Autodesk Fusion 360 part; units mm, degrees
(part 11 of 12)
  spline S88 degree 5 poles (70.3993, -3.7669) (70.38, -3.7562) (70.3415, -3.7349) (70.2837, -3.7032) (70.2065, -3.661) (70.1099, -3.6088) (70.0133, -3.5569) (69.9165, -3.5054) (69.8196, -3.4543) (69.7226, -3.4037) (69.6255, -3.3534) (69.5283, -3.3036) (69.431, -3.2541) (69.3336, -3.2051) (69.2361, -3.1565) (69.1385, -3.1083) (69.0408, -3.0606) (68.943, -3.0133) (68.8451, -2.9664) (68.747, -2.9199) (68.6489, -2.8739) (68.5507, -2.8284) (68.4524, -2.7832) (68.3539, -2.7386) (68.2554, -2.6944) (68.1568, -2.6506) (68.0581, -2.6073) (67.9593, -2.5645) (67.8604, -2.5221) (67.7613, -2.4803) (67.6622, -2.4389) (67.563, -2.398) (67.4637, -2.3575) (67.3643, -2.3176) (67.2649, -2.2782) (67.1653, -2.2393) (67.0656, -2.2009) (66.9658, -2.1631) (66.866, -2.1257) (66.766, -2.0889) (66.6659, -2.0527) (66.5658, -2.0169) (66.4656, -1.9818) (66.3652, -1.9472) (66.2648, -1.9132) (66.1643, -1.8797) (66.0637, -1.8469) (65.963, -1.8147) (65.8622, -1.7831) (65.7614, -1.7521) (65.6604, -1.7217) (65.5593, -1.692) (65.4582, -1.663) (65.357, -1.6346) (65.2557, -1.6069) (65.1614, -1.5819) (65.0873, -1.5627) (65.0336, -1.5491) (65.0001, -1.5407) (64.9869, -1.5374) knots -1 -1 -1 -1 -1 -1 -0.985714 -0.971429 -0.957143 -0.942857 -0.928571 -0.914286 -0.9 -0.885714 -0.871429 -0.857143 -0.842857 -0.828571 -0.814286 -0.8 -0.785714 -0.771429 -0.757143 -0.742857 -0.728571 -0.714286 -0.7 -0.685714 -0.671429 -0.657143 -0.642857 -0.628571 -0.614286 -0.6 -0.585714 -0.571429 -0.557143 -0.542857 -0.528571 -0.514286 -0.5 -0.485714 -0.471429 -0.457143 -0.442857 -0.428571 -0.414286 -0.4 -0.385714 -0.371429 -0.357143 -0.342857 -0.328571 -0.314286 -0.3 -0.285714 -0.271429 -0.257143 -0.242857 -0.228571 -0.21931 -0.21931 -0.21931 -0.21931 -0.21931 -0.21931
  spline S89 degree 3 poles (64.9869, -1.5374) (64.7974, -1.4903) (64.6188, -1.4065) (64.304, -1.1753) (64.1706, -1.0301) (63.9972, -0.746) (63.942, -0.6193) (63.8677, -0.3544) (63.849, -0.2175) (63.8491, -0.0799) knots 0 0 0 0 0.058597 0.058597 0.117193 0.117193 0.158456 0.158456 0.199718 0.199718 0.199718 0.199718
  arc A45 (63.8491, -0.0799) -> (63.8491, 0.0799) centre (0, 0) ccw
  spline S90 degree 3 poles (63.8491, 0.0799) (63.8489, 0.2753) (63.8868, 0.4688) (64.0347, 0.8304) (64.1432, 0.995) (64.3767, 1.2322) (64.4862, 1.3165) (64.7252, 1.4528) (64.8534, 1.5042) (64.9869, 1.5374) knots 0 0 0 0 0.058597 0.058597 0.117193 0.117193 0.158456 0.158456 0.199718 0.199718 0.199718 0.199718
  spline S91 degree 5 poles (64.9869, 1.5374) (65.0001, 1.5407) (65.0336, 1.5491) (65.0873, 1.5627) (65.1614, 1.5819) (65.2557, 1.6069) (65.357, 1.6346) (65.4582, 1.663) (65.5593, 1.692) (65.6604, 1.7217) (65.7614, 1.7521) (65.8622, 1.7831) (65.963, 1.8147) (66.0637, 1.8469) (66.1643, 1.8797) (66.2648, 1.9132) (66.3652, 1.9472) (66.4656, 1.9818) (66.5658, 2.0169) (66.6659, 2.0527) (66.766, 2.0889) (66.866, 2.1257) (66.9658, 2.1631) (67.0656, 2.2009) (67.1653, 2.2393) (67.2649, 2.2782) (67.3643, 2.3176) (67.4637, 2.3575) (67.563, 2.398) (67.6622, 2.4389) (67.7613, 2.4803) (67.8604, 2.5221) (67.9593, 2.5645) (68.0581, 2.6073) (68.1568, 2.6506) (68.2554, 2.6944) (68.3539, 2.7386) (68.4524, 2.7832) (68.5507, 2.8284) (68.6489, 2.8739) (68.747, 2.9199) (68.8451, 2.9664) (68.943, 3.0133) (69.0408, 3.0606) (69.1385, 3.1083) (69.2361, 3.1565) (69.3336, 3.2051) (69.431, 3.2541) (69.5283, 3.3036) (69.6255, 3.3534) (69.7226, 3.4037) (69.8196, 3.4543) (69.9165, 3.5054) (70.0133, 3.5569) (70.1099, 3.6088) (70.2065, 3.661) (70.2837, 3.7032) (70.3415, 3.7349) (70.38, 3.7562) (70.3993, 3.7669) knots 0.21931 0.21931 0.21931 0.21931 0.21931 0.21931 0.228571 0.242857 0.257143 0.271429 0.285714 0.3 0.314286 0.328571 0.342857 0.357143 0.371429 0.385714 0.4 0.414286 0.428571 0.442857 0.457143 0.471429 0.485714 0.5 0.514286 0.528571 0.542857 0.557143 0.571429 0.585714 0.6 0.614286 0.628571 0.642857 0.657143 0.671429 0.685714 0.7 0.714286 0.728571 0.742857 0.757143 0.771429 0.785714 0.8 0.814286 0.828571 0.842857 0.857143 0.871429 0.885714 0.9 0.914286 0.928571 0.942857 0.957143 0.971429 0.985714 1 1 1 1 1 1
  arc A46 (70.3993, 3.7669) -> (70.2384, 6.0675) centre (0, 0) ccw
  spline S92 degree 5 poles (70.2384, 6.0675) (70.2179, 6.0754) (70.1768, 6.0911) (70.1151, 6.1145) (70.0328, 6.1455) (69.9299, 6.1838) (69.8269, 6.2217) (69.7239, 6.2592) (69.6209, 6.2963) (69.5178, 6.333) (69.4147, 6.3692) (69.3115, 6.4051) (69.2082, 6.4405) (69.1049, 6.4755) (69.0016, 6.51) (68.8983, 6.5441) (68.7948, 6.5778) (68.6914, 6.6111) (68.5879, 6.6439) (68.4844, 6.6762) (68.3808, 6.7081) (68.2772, 6.7396) (68.1735, 6.7706) (68.0699, 6.8011) (67.9662, 6.8312) (67.8624, 6.8608) (67.7586, 6.8899) (67.6548, 6.9186) (67.551, 6.9467) (67.4471, 6.9744) (67.3432, 7.0016) (67.2393, 7.0283) (67.1353, 7.0545) (67.0313, 7.0802) (66.9273, 7.1054) (66.8233, 7.1301) (66.7192, 7.1542) (66.6152, 7.1778) (66.5111, 7.2009) (66.407, 7.2234) (66.3028, 7.2454) (66.1987, 7.2669) (66.0945, 7.2877) (65.9904, 7.308) (65.8862, 7.3277) (65.782, 7.3469) (65.6778, 7.3654) (65.5736, 7.3833) (65.4694, 7.4005) (65.3652, 7.4172) (65.261, 7.4332) (65.1568, 7.4485) (65.0526, 7.4632) (64.9484, 7.4772) (64.8442, 7.4905) (64.7474, 7.5022) (64.6714, 7.5109) (64.6163, 7.5169) (64.5819, 7.5205) (64.5684, 7.522) knots -1 -1 -1 -1 -1 -1 -0.985714 -0.971429 -0.957143 -0.942857 -0.928571 -0.914286 -0.9 -0.885714 -0.871429 -0.857143 -0.842857 -0.828571 -0.814286 -0.8 -0.785714 -0.771429 -0.757143 -0.742857 -0.728571 -0.714286 -0.7 -0.685714 -0.671429 -0.657143 -0.642857 -0.628571 -0.614286 -0.6 -0.585714 -0.571429 -0.557143 -0.542857 -0.528571 -0.514286 -0.5 -0.485714 -0.471429 -0.457143 -0.442857 -0.428571 -0.414286 -0.4 -0.385714 -0.371429 -0.357143 -0.342857 -0.328571 -0.314286 -0.3 -0.285714 -0.271429 -0.257143 -0.242857 -0.228571 -0.21931 -0.21931 -0.21931 -0.21931 -0.21931 -0.21931
  spline S93 degree 3 poles (64.5684, 7.522) (64.3742, 7.5423) (64.1857, 7.6004) (63.8417, 7.7855) (63.6895, 7.9108) (63.4782, 8.168) (63.4059, 8.2858) (63.2955, 8.5377) (63.2579, 8.6707) (63.2389, 8.8069) knots 0 0 0 0 0.058597 0.058597 0.117193 0.117193 0.158456 0.158456 0.199718 0.199718 0.199718 0.199718
  arc A47 (63.2389, 8.8069) -> (63.2166, 8.9653) centre (0, 0) ccw
  spline S94 degree 3 poles (63.2166, 8.9653) (63.1892, 9.1586) (63.1998, 9.3555) (63.2959, 9.7342) (63.3805, 9.9123) (63.5787, 10.1797) (63.6755, 10.2784) (63.8931, 10.4467) (64.0129, 10.5154) (64.1405, 10.5669) knots 0 0 0 0 0.058597 0.058597 0.117193 0.117193 0.158456 0.158456 0.199718 0.199718 0.199718 0.199718
  spline S95 degree 5 poles (64.1405, 10.5669) (64.1531, 10.572) (64.1851, 10.5849) (64.2364, 10.6059) (64.3071, 10.6352) (64.397, 10.6731) (64.4934, 10.7146) (64.5897, 10.7568) (64.6858, 10.7997) (64.7818, 10.8432) (64.8775, 10.8873) (64.9731, 10.932) (65.0685, 10.9773) (65.1637, 11.0232) (65.2588, 11.0697) (65.3537, 11.1168) (65.4484, 11.1645) (65.5429, 11.2127) (65.6373, 11.2615) (65.7315, 11.3108) (65.8255, 11.3606) (65.9194, 11.411) (66.0131, 11.4618) (66.1066, 11.5132) (66.2, 11.5651) (66.2932, 11.6175) (66.3862, 11.6704) (66.4791, 11.7237) (66.5718, 11.7776) (66.6643, 11.8319) (66.7567, 11.8867) (66.8489, 11.9419) (66.941, 11.9976) (67.0329, 12.0538) (67.1246, 12.1104) (67.2162, 12.1675) (67.3076, 12.225) (67.3988, 12.2829) (67.4899, 12.3412) (67.5809, 12.4) (67.6716, 12.4593) (67.7622, 12.5189) (67.8527, 12.579) (67.9429, 12.6394) (68.0331, 12.7003) (68.123, 12.7616) (68.2128, 12.8233) (68.3024, 12.8854) (68.3919, 12.9479) (68.4812, 13.0108) (68.5704, 13.0741) (68.6594, 13.1377) (68.7482, 13.2018) (68.8369, 13.2662) (68.9254, 13.3311) (69.0138, 13.3963) (69.0843, 13.4487) (69.1371, 13.4882) (69.1723, 13.5147) (69.1899, 13.5279) knots 0.21931 0.21931 0.21931 0.21931 0.21931 0.21931 0.228571 0.242857 0.257143 0.271429 0.285714 0.3 0.314286 0.328571 0.342857 0.357143 0.371429 0.385714 0.4 0.414286 0.428571 0.442857 0.457143 0.471429 0.485714 0.5 0.514286 0.528571 0.542857 0.557143 0.571429 0.585714 0.6 0.614286 0.628571 0.642857 0.657143 0.671429 0.685714 0.7 0.714286 0.728571 0.742857 0.757143 0.771429 0.785714 0.8 0.814286 0.828571 0.842857 0.857143 0.871429 0.885714 0.9 0.914286 0.928571 0.942857 0.957143 0.971429 0.985714 1 1 1 1 1 1
  arc A48 (69.1899, 13.5279) -> (68.7104, 15.7837) centre (0, 0) ccw
  spline S96 degree 5 poles (68.7104, 15.7837) (68.689, 15.7887) (68.6461, 15.7985) (68.5817, 15.8131) (68.4959, 15.8323) (68.3887, 15.856) (68.2815, 15.8792) (68.1743, 15.902) (68.0671, 15.9244) (67.9599, 15.9463) (67.8527, 15.9679) (67.7455, 15.989) (67.6384, 16.0097) (67.5312, 16.03) (67.4241, 16.0498) (67.317, 16.0692) (67.2099, 16.0882) (67.1028, 16.1067) (66.9958, 16.1248) (66.8887, 16.1424) (66.7817, 16.1596) (66.6748, 16.1763) (66.5678, 16.1926) (66.4609, 16.2084) (66.354, 16.2238) (66.2471, 16.2386) (66.1403, 16.253) (66.0335, 16.267) (65.9268, 16.2804) (65.82, 16.2934) (65.7134, 16.3059) (65.6067, 16.3178) (65.5001, 16.3293) (65.3936, 16.3403) (65.2871, 16.3507) (65.1806, 16.3607) (65.0742, 16.3701) (64.9679, 16.379) (64.8616, 16.3874) (64.7554, 16.3952) (64.6492, 16.4025) (64.5431, 16.4092) (64.4371, 16.4154) (64.3311, 16.421) (64.2252, 16.426) (64.1193, 16.4304) (64.0136, 16.4343) (63.9079, 16.4375) (63.8023, 16.4401) (63.6968, 16.4421) (63.5914, 16.4434) (63.4861, 16.4441) (63.3809, 16.4442) (63.2757, 16.4435) (63.1707, 16.4422) (63.0732, 16.4403) (62.9967, 16.4383) (62.9413, 16.4366) (62.9068, 16.4354) (62.8932, 16.4349) knots -1 -1 -1 -1 -1 -1 -0.985714 -0.971429 -0.957143 -0.942857 -0.928571 -0.914286 -0.9 -0.885714 -0.871429 -0.857143 -0.842857 -0.828571 -0.814286 -0.8 -0.785714 -0.771429 -0.757143 -0.742857 -0.728571 -0.714286 -0.7 -0.685714 -0.671429 -0.657143 -0.642857 -0.628571 -0.614286 -0.6 -0.585714 -0.571429 -0.557143 -0.542857 -0.528571 -0.514286 -0.5 -0.485714 -0.471429 -0.457143 -0.442857 -0.428571 -0.414286 -0.4 -0.385714 -0.371429 -0.357143 -0.342857 -0.328571 -0.314286 -0.3 -0.285714 -0.271429 -0.257143 -0.242857 -0.228571 -0.21931 -0.21931 -0.21931 -0.21931 -0.21931 -0.21931
  spline S97 degree 3 poles (62.8932, 16.4349) (62.698, 16.428) (62.5033, 16.4593) (62.1369, 16.5948) (61.9687, 16.6976) (61.7237, 16.9229) (61.6357, 17.0295) (61.4913, 17.2637) (61.4355, 17.3901) (61.3978, 17.5224) knots 0 0 0 0 0.058597 0.058597 0.117193 0.117193 0.158456 0.158456 0.199718 0.199718 0.199718 0.199718
  arc A49 (61.3978, 17.5224) -> (61.3537, 17.6761) centre (0, 0) ccw
  spline S98 degree 3 poles (61.3537, 17.6761) (61.2996, 17.8638) (61.2827, 18.0602) (61.3252, 18.4485) (61.3842, 18.6367) (61.5432, 18.9291) (61.6253, 19.0403) (61.8174, 19.2372) (61.9265, 19.322) (62.0457, 19.3907) knots 0 0 0 0 0.058597 0.058597 0.117193 0.117193 0.158456 0.158456 0.199718 0.199718 0.199718 0.199718
  spline S99 degree 5 poles (62.0457, 19.3907) (62.0574, 19.3975) (62.0873, 19.4148) (62.1352, 19.4427) (62.2011, 19.4815) (62.2848, 19.5316) (62.3746, 19.5861) (62.4641, 19.6413) (62.5533, 19.6971) (62.6422, 19.7535) (62.7309, 19.8105) (62.8194, 19.8681) (62.9075, 19.9262) (62.9954, 19.985) (63.0831, 20.0443) (63.1705, 20.1041) (63.2576, 20.1645) (63.3445, 20.2254) (63.4312, 20.2868) (63.5176, 20.3488) (63.6038, 20.4112) (63.6898, 20.4741) (63.7755, 20.5375) (63.8609, 20.6014) (63.9462, 20.6658) (64.0312, 20.7307) (64.1159, 20.796) (64.2005, 20.8617) (64.2848, 20.928) (64.3689, 20.9946) (64.4527, 21.0617) (64.5364, 21.1293) (64.6198, 21.1973) (64.703, 21.2657) (64.7859, 21.3345) (64.8687, 21.4037) (64.9512, 21.4734) (65.0335, 21.5435) (65.1155, 21.6139) (65.1974, 21.6848) (65.279, 21.7561) (65.3605, 21.8277) (65.4417, 21.8998) (65.5227, 21.9723) (65.6034, 22.0451) (65.684, 22.1183) (65.7643, 22.1919) (65.8444, 22.2659) (65.9243, 22.3402) (66.004, 22.4149) (66.0835, 22.49) (66.1628, 22.5654) (66.2418, 22.6412) (66.3207, 22.7174) (66.3993, 22.7939) (66.4777, 22.8707) (66.5403, 22.9325) (66.5871, 22.979) (66.6183, 23.0101) (66.6339, 23.0256) knots 0.21931 0.21931 0.21931 0.21931 0.21931 0.21931 0.228571 0.242857 0.257143 0.271429 0.285714 0.3 0.314286 0.328571 0.342857 0.357143 0.371429 0.385714 0.4 0.414286 0.428571 0.442857 0.457143 0.471429 0.485714 0.5 0.514286 0.528571 0.542857 0.557143 0.571429 0.585714 0.6 0.614286 0.628571 0.642857 0.657143 0.671429 0.685714 0.7 0.714286 0.728571 0.742857 0.757143 0.771429 0.785714 0.8 0.814286 0.828571 0.842857 0.857143 0.871429 0.885714 0.9 0.914286 0.928571 0.942857 0.957143 0.971429 0.985714 1 1 1 1 1 1
  arc A50 (66.6339, 23.0256) -> (65.8451, 25.1928) centre (0, 0) ccw
  spline S100 degree 5 poles (65.8451, 25.1928) (65.8231, 25.1947) (65.7793, 25.1984) (65.7135, 25.2039) (65.6259, 25.211) (65.5164, 25.2195) (65.407, 25.2276) (65.2977, 25.2352) (65.1884, 25.2425) (65.0792, 25.2493) (64.9701, 25.2558) (64.861, 25.2618) (64.752, 25.2673) (64.6431, 25.2725) (64.5342, 25.2772) (64.4254, 25.2815) (64.3168, 25.2854) (64.2081, 25.2889) (64.0996, 25.2919) (63.9912, 25.2944) (63.8828, 25.2966) (63.7746, 25.2982) (63.6664, 25.2995) (63.5583, 25.3002) (63.4503, 25.3006) (63.3424, 25.3004) (63.2346, 25.2998) (63.127, 25.2988) (63.0194, 25.2972) (62.9119, 25.2952) (62.8045, 25.2927) (62.6972, 25.2897) (62.5901, 25.2862) (62.4831, 25.2823) (62.3761, 25.2778) (62.2693, 25.2729) (62.1627, 25.2674) (62.0561, 25.2614) (61.9497, 25.2549) (61.8434, 25.2479) (61.7373, 25.2403) (61.6312, 25.2322) (61.5254, 25.2235) (61.4197, 25.2143) (61.3141, 25.2046) (61.2087, 25.1942) (61.1034, 25.1833) (60.9983, 25.1718) (60.8934, 25.1597) (60.7886, 25.1469) (60.6841, 25.1336) (60.5797, 25.1196) (60.4755, 25.105) (60.3714, 25.0898) (60.2676, 25.0739) (60.1713, 25.0584) (60.0959, 25.0458) (60.0412, 25.0364) (60.0072, 25.0304) (59.9938, 25.028) knots -1 -1 -1 -1 -1 -1 -0.985714 -0.971429 -0.957143 -0.942857 -0.928571 -0.914286 -0.9 -0.885714 -0.871429 -0.857143 -0.842857 -0.828571 -0.814286 -0.8 -0.785714 -0.771429 -0.757143 -0.742857 -0.728571 -0.714286 -0.7 -0.685714 -0.671429 -0.657143 -0.642857 -0.628571 -0.614286 -0.6 -0.585714 -0.571429 -0.557143 -0.542857 -0.528571 -0.514286 -0.5 -0.485714 -0.471429 -0.457143 -0.442857 -0.428571 -0.414286 -0.4 -0.385714 -0.371429 -0.357143 -0.342857 -0.328571 -0.314286 -0.3 -0.285714 -0.271429 -0.257143 -0.242857 -0.228571 -0.21931 -0.21931 -0.21931 -0.21931 -0.21931 -0.21931
  spline S101 degree 3 poles (59.9938, 25.028) (59.8015, 24.994) (59.6043, 24.9979) (59.2226, 25.0811) (59.0417, 25.1595) (58.7677, 25.3485) (58.6658, 25.4418) (58.4902, 25.6536) (58.4174, 25.771) (58.3616, 25.8968) knots 0 0 0 0 0.058597 0.058597 0.117193 0.117193 0.158456 0.158456 0.199718 0.199718 0.199718 0.199718
  arc A51 (58.3616, 25.8968) -> (58.2966, 26.0428) centre (0, 0) ccw
  spline S102 degree 3 poles (58.2966, 26.0428) (58.2169, 26.2212) (58.1728, 26.4134) (58.1608, 26.8038) (58.193, 26.9983) (58.3099, 27.31) (58.3757, 27.4316) (58.5385, 27.6533) (58.6347, 27.7524) (58.7432, 27.8371) knots 0 0 0 0 0.058597 0.058597 0.117193 0.117193 0.158456 0.158456 0.199718 0.199718 0.199718 0.199718
  spline S103 degree 5 poles (58.7432, 27.8371) (58.7539, 27.8454) (58.781, 27.8667) (58.8246, 27.901) (58.8845, 27.9486) (58.9604, 28.0099) (59.0417, 28.0764) (59.1226, 28.1435) (59.2032, 28.2111) (59.2835, 28.2794) (59.3634, 28.3482) (59.4429, 28.4175) (59.5221, 28.4874) (59.601, 28.5578) (59.6795, 28.6287) (59.7578, 28.7001) (59.8357, 28.772) (59.9133, 28.8444) (59.9905, 28.9173) (60.0675, 28.9907) (60.1441, 29.0645) (60.2205, 29.1388) (60.2965, 29.2135) (60.3723, 29.2887) (60.4477, 29.3643) (60.5229, 29.4403) (60.5977, 29.5168) (60.6723, 29.5937) (60.7466, 29.671) (60.8206, 29.7487) (60.8943, 29.8269) (60.9677, 29.9054) (61.0408, 29.9843) (61.1137, 30.0636) (61.1862, 30.1433) (61.2585, 30.2234) (61.3306, 30.3039) (61.4023, 30.3847) (61.4738, 30.4659) (61.545, 30.5475) (61.6159, 30.6294) (61.6865, 30.7117) (61.7569, 30.7944) (61.827, 30.8774) (61.8969, 30.9608) (61.9665, 31.0445) (62.0358, 31.1285) (62.1048, 31.2129) (62.1736, 31.2977) (62.2421, 31.3828) (62.3104, 31.4682) (62.3784, 31.5539) (62.4461, 31.64) (62.5136, 31.7263) (62.5808, 31.813) (62.6478, 31.9001) (62.7011, 31.97) (62.741, 32.0225) (62.7676, 32.0576) (62.7808, 32.0752) knots 0.21931 0.21931 0.21931 0.21931 0.21931 0.21931 0.228571 0.242857 0.257143 0.271429 0.285714 0.3 0.314286 0.328571 0.342857 0.357143 0.371429 0.385714 0.4 0.414286 0.428571 0.442857 0.457143 0.471429 0.485714 0.5 0.514286 0.528571 0.542857 0.557143 0.571429 0.585714 0.6 0.614286 0.628571 0.642857 0.657143 0.671429 0.685714 0.7 0.714286 0.728571 0.742857 0.757143 0.771429 0.785714 0.8 0.814286 0.828571 0.842857 0.857143 0.871429 0.885714 0.9 0.914286 0.928571 0.942857 0.957143 0.971429 0.985714 1 1 1 1 1 1
  arc A52 (62.7808, 32.0752) -> (61.6981, 34.1115) centre (0, 0) ccw
  spline S104 degree 5 poles (61.6981, 34.1115) (61.6761, 34.1103) (61.6322, 34.1079) (61.5663, 34.1042) (61.4785, 34.0991) (61.369, 34.0922) (61.2595, 34.085) (61.1501, 34.0773) (61.0409, 34.0693) (60.9318, 34.0609) (60.8228, 34.0521) (60.714, 34.0428) (60.6053, 34.0332) (60.4967, 34.0231) (60.3883, 34.0127) (60.2799, 34.0018) (60.1718, 33.9905) (60.0637, 33.9788) (59.9559, 33.9667) (59.8481, 33.9541) (59.7405, 33.9411) (59.6331, 33.9277) (59.5258, 33.9139) (59.4187, 33.8996) (59.3117, 33.8849) (59.2049, 33.8698) (59.0982, 33.8542) (58.9917, 33.8381) (58.8854, 33.8216) (58.7792, 33.8047) (58.6732, 33.7872) (58.5674, 33.7694) (58.4618, 33.751) (58.3564, 33.7322) (58.2511, 33.7129) (58.146, 33.6931) (58.0412, 33.6729) (57.9365, 33.6521) (57.832, 33.6308) (57.7277, 33.6091) (57.6237, 33.5868) (57.5198, 33.564) (57.4162, 33.5407) (57.3128, 33.5169) (57.2096, 33.4925) (57.1066, 33.4676) (57.0039, 33.4422) (56.9014, 33.4161) (56.7992, 33.3895) (56.6973, 33.3624) (56.5956, 33.3346) (56.4941, 33.3062) (56.393, 33.2773) (56.2921, 33.2477) (56.1915, 33.2175) (56.0983, 33.1888) (56.0253, 33.1658) (55.9725, 33.1488) (55.9396, 33.1382) (55.9267, 33.134) knots -1 -1 -1 -1 -1 -1 -0.985714 -0.971429 -0.957143 -0.942857 -0.928571 -0.914286 -0.9 -0.885714 -0.871429 -0.857143 -0.842857 -0.828571 -0.814286 -0.8 -0.785714 -0.771429 -0.757143 -0.742857 -0.728571 -0.714286 -0.7 -0.685714 -0.671429 -0.657143 -0.642857 -0.628571 -0.614286 -0.6 -0.585714 -0.571429 -0.557143 -0.542857 -0.528571 -0.514286 -0.5 -0.485714 -0.471429 -0.457143 -0.442857 -0.428571 -0.414286 -0.4 -0.385714 -0.371429 -0.357143 -0.342857 -0.328571 -0.314286 -0.3 -0.285714 -0.271429 -0.257143 -0.242857 -0.228571 -0.21931 -0.21931 -0.21931 -0.21931 -0.21931 -0.21931
  spline S105 degree 3 poles (55.9267, 33.134) (55.741, 33.0736) (55.5452, 33.05) (55.1557, 33.0792) (54.9656, 33.1317) (54.668, 33.2807) (54.5541, 33.3589) (54.3507, 33.5442) (54.2623, 33.6504) (54.1895, 33.7671) knots 0 0 0 0 0.058597 0.058597 0.117193 0.117193 0.158456 0.158456 0.199718 0.199718 0.199718 0.199718
  arc A53 (54.1895, 33.7671) -> (54.1048, 33.9027) centre (0, 0) ccw
  spline S106 degree 3 poles (54.1048, 33.9027) (54.0011, 34.0682) (53.9307, 34.2524) (53.8645, 34.6374) (53.8693, 34.8345) (53.9416, 35.1594) (53.9898, 35.2889) (54.1202, 35.5312) (54.2017, 35.6427) (54.2973, 35.7416) knots 0 0 0 0 0.058597 0.058597 0.117193 0.117193 0.158456 0.158456 0.199718 0.199718 0.199718 0.199718
  spline S107 degree 5 poles (54.2973, 35.7416) (54.3067, 35.7514) (54.3307, 35.7762) (54.3691, 35.8163) (54.4217, 35.8718) (54.4884, 35.943) (54.5597, 36.0202) (54.6305, 36.0979) (54.7008, 36.1761) (54.7708, 36.2548) (54.8403, 36.3341) (54.9095, 36.4138) (54.9782, 36.494) (55.0465, 36.5747) (55.1144, 36.6558) (55.1819, 36.7375) (55.2491, 36.8195) (55.3158, 36.902) (55.3822, 36.985) (55.4482, 37.0683) (55.5138, 37.1521) (55.5791, 37.2363) (55.644, 37.3209) (55.7085, 37.4058) (55.7727, 37.4912) (55.8366, 37.577) (55.9, 37.6631) (55.9632, 37.7496) (56.026, 37.8365) (56.0884, 37.9238) (56.1505, 38.0114) (56.2123, 38.0994) (56.2738, 38.1877) (56.3349, 38.2764) (56.3956, 38.3654) (56.4561, 38.4548) (56.5162, 38.5445) (56.576, 38.6346) (56.6355, 38.7249) (56.6946, 38.8156) (56.7535, 38.9066) (56.812, 38.998) (56.8702, 39.0896) (56.928, 39.1816) (56.9856, 39.2739) (57.0429, 39.3664) (57.0998, 39.4593) (57.1564, 39.5525) (57.2127, 39.646) (57.2688, 39.7398) (57.3245, 39.8338) (57.3799, 39.9282) (57.435, 40.0229) (57.4898, 40.1178) (57.5443, 40.213) (57.5985, 40.3085) (57.6416, 40.3851) (57.6738, 40.4427) (57.6952, 40.4812) (57.7059, 40.5004) knots 0.21931 0.21931 0.21931 0.21931 0.21931 0.21931 0.228571 0.242857 0.257143 0.271429 0.285714 0.3 0.314286 0.328571 0.342857 0.357143 0.371429 0.385714 0.4 0.414286 0.428571 0.442857 0.457143 0.471429 0.485714 0.5 0.514286 0.528571 0.542857 0.557143 0.571429 0.585714 0.6 0.614286 0.628571 0.642857 0.657143 0.671429 0.685714 0.7 0.714286 0.728571 0.742857 0.757143 0.771429 0.785714 0.8 0.814286 0.828571 0.842857 0.857143 0.871429 0.885714 0.9 0.914286 0.928571 0.942857 0.957143 0.971429 0.985714 1 1 1 1 1 1
  arc A54 (57.7059, 40.5004) -> (56.3503, 42.3662) centre (0, 0) ccw
  spline S108 degree 5 poles (56.3503, 42.3662) (56.3287, 42.362) (56.2855, 42.3535) (56.2208, 42.3407) (56.1346, 42.3234) (56.027, 42.3013) (55.9196, 42.2789) (55.8124, 42.2562) (55.7053, 42.233) (55.5985, 42.2095) (55.4918, 42.1856) (55.3853, 42.1613) (55.279, 42.1366) (55.1729, 42.1115) (55.0669, 42.0861) (54.9612, 42.0602) (54.8556, 42.034) (54.7503, 42.0074) (54.6451, 41.9804) (54.5402, 41.9529) (54.4354, 41.9251) (54.3309, 41.8969) (54.2266, 41.8682) (54.1225, 41.8392) (54.0186, 41.8097) (53.9149, 41.7799) (53.8115, 41.7496) (53.7082, 41.7189) (53.6052, 41.6877) (53.5025, 41.6562) (53.4, 41.6242) (53.2977, 41.5917) (53.1956, 41.5589) (53.0938, 41.5256) (52.9923, 41.4918) (52.891, 41.4576) (52.79, 41.4229) (52.6892, 41.3878) (52.5887, 41.3522) (52.4884, 41.3162) (52.3885, 41.2796) (52.2888, 41.2426) (52.1894, 41.2051) (52.0903, 41.1671) (51.9916, 41.1286) (51.8931, 41.0896) (51.7949, 41.0501) (51.697, 41.0101) (51.5995, 40.9695) (51.5023, 40.9284) (51.4055, 40.8868) (51.309, 40.8446) (51.2129, 40.8018) (51.1171, 40.7585) (51.0217, 40.7146) (50.9333, 40.6731) (50.8643, 40.6402) (50.8143, 40.6161) (50.7833, 40.601) (50.7711, 40.595) knots -1 -1 -1 -1 -1 -1 -0.985714 -0.971429 -0.957143 -0.942857 -0.928571 -0.914286 -0.9 -0.885714 -0.871429 -0.857143 -0.842857 -0.828571 -0.814286 -0.8 -0.785714 -0.771429 -0.757143 -0.742857 -0.728571 -0.714286 -0.7 -0.685714 -0.671429 -0.657143 -0.642857 -0.628571 -0.614286 -0.6 -0.585714 -0.571429 -0.557143 -0.542857 -0.528571 -0.514286 -0.5 -0.485714 -0.471429 -0.457143 -0.442857 -0.428571 -0.414286 -0.4 -0.385714 -0.371429 -0.357143 -0.342857 -0.328571 -0.314286 -0.3 -0.285714 -0.271429 -0.257143 -0.242857 -0.228571 -0.21931 -0.21931 -0.21931 -0.21931 -0.21931 -0.21931
  spline S109 degree 3 poles (50.7711, 40.595) (50.5956, 40.5093) (50.405, 40.4587) (50.0152, 40.4334) (49.8197, 40.459) (49.5042, 40.5651) (49.3805, 40.6267) (49.1533, 40.7819) (49.051, 40.8747) (48.9627, 40.9802) knots 0 0 0 0 0.058597 0.058597 0.117193 0.117193 0.158456 0.158456 0.199718 0.199718 0.199718 0.199718
  arc A55 (48.9627, 40.9802) -> (48.8599, 41.1027) centre (0, 0) ccw
  spline S110 degree 3 poles (48.8599, 41.1027) (48.7342, 41.2522) (48.6388, 41.4248) (48.5197, 41.7968) (48.497, 41.9927) (48.5234, 42.3245) (48.5531, 42.4594) (48.6485, 42.7174) (48.7137, 42.8393) (48.7946, 42.9505) knots 0 0 0 0 0.058597 0.058597 0.117193 0.117193 0.158456 0.158456 0.199718 0.199718 0.199718 0.199718
  spline S111 degree 5 poles (48.7946, 42.9505) (48.8026, 42.9615) (48.8229, 42.9894) (48.8553, 43.0345) (48.8997, 43.0967) (48.9558, 43.1765) (49.0156, 43.2629) (49.0749, 43.3497) (49.1338, 43.4369) (49.1921, 43.5246) (49.2499, 43.6128) (49.3073, 43.7013) (49.3642, 43.7903) (49.4206, 43.8797) (49.4765, 43.9696) (49.532, 44.0598) (49.5871, 44.1504) (49.6417, 44.2414) (49.6959, 44.3327) (49.7497, 44.4245) (49.803, 44.5166) (49.8559, 44.609) (49.9084, 44.7018) (49.9605, 44.7949) (50.0122, 44.8884) (50.0635, 44.9822) (50.1143, 45.0764) (50.1648, 45.1708) (50.2149, 45.2656) (50.2646, 45.3607) (50.3139, 45.4561) (50.3629, 45.5519) (50.4114, 45.6479) (50.4596, 45.7442) (50.5074, 45.8408) (50.5548, 45.9377) (50.6018, 46.0349) (50.6485, 46.1324) (50.6948, 46.2302) (50.7408, 46.3282) (50.7864, 46.4265) (50.8316, 46.5251) (50.8765, 46.624) (50.921, 46.7231) (50.9652, 46.8225) (51.009, 46.9222) (51.0524, 47.0221) (51.0955, 47.1222) (51.1383, 47.2226) (51.1807, 47.3233) (51.2228, 47.4242) (51.2645, 47.5254) (51.3059, 47.6268) (51.347, 47.7284) (51.3877, 47.8303) (51.428, 47.9324) (51.4601, 48.0143) (51.4839, 48.0758) (51.4998, 48.1168) (51.5077, 48.1374) knots 0.21931 0.21931 0.21931 0.21931 0.21931 0.21931 0.228571 0.242857 0.257143 0.271429 0.285714 0.3 0.314286 0.328571 0.342857 0.357143 0.371429 0.385714 0.4 0.414286 0.428571 0.442857 0.457143 0.471429 0.485714 0.5 0.514286 0.528571 0.542857 0.557143 0.571429 0.585714 0.6 0.614286 0.628571 0.642857 0.657143 0.671429 0.685714 0.7 0.714286 0.728571 0.742857 0.757143 0.771429 0.785714 0.8 0.814286 0.828571 0.842857 0.857143 0.871429 0.885714 0.9 0.914286 0.928571 0.942857 0.957143 0.971429 0.985714 1 1 1 1 1 1
  arc A56 (51.5077, 48.1374) -> (49.9056, 49.7964) centre (0, 0) ccw
  spline S112 degree 5 poles (49.9056, 49.7964) (49.8848, 49.7892) (49.8433, 49.7748) (49.7809, 49.7531) (49.698, 49.7239) (49.5945, 49.6871) (49.4913, 49.65) (49.3883, 49.6125) (49.2855, 49.5747) (49.183, 49.5365) (49.0807, 49.498) (48.9786, 49.4591) (48.8767, 49.4199) (48.7751, 49.3803) (48.6738, 49.3403) (48.5726, 49.3) (48.4718, 49.2594) (48.3712, 49.2183) (48.2708, 49.1769) (48.1707, 49.1352) (48.0708, 49.093) (47.9712, 49.0505) (47.8719, 49.0077) (47.7729, 48.9644) (47.6741, 48.9208) (47.5756, 48.8768) (47.4774, 48.8324) (47.3794, 48.7876) (47.2818, 48.7424) (47.1844, 48.6969) (47.0873, 48.6509) (46.9905, 48.6046) (46.8941, 48.5578) (46.7979, 48.5107) (46.702, 48.4631) (46.6065, 48.4151) (46.5112, 48.3667) (46.4163, 48.3179) (46.3218, 48.2687) (46.2275, 48.219) (46.1336, 48.169) (46.0401, 48.1184) (45.9469, 48.0675) (45.8541, 48.0161) (45.7616, 47.9642) (45.6695, 47.9119) (45.5778, 47.8591) (45.4864, 47.8058) (45.3955, 47.7521) (45.305, 47.6978) (45.2149, 47.6431) (45.1252, 47.5879) (45.0359, 47.5322) (44.9471, 47.4759) (44.8588, 47.4192) (44.7771, 47.3659) (44.7133, 47.3237) (44.6671, 47.2928) (44.6385, 47.2735) (44.6273, 47.2659) knots -1 -1 -1 -1 -1 -1 -0.985714 -0.971429 -0.957143 -0.942857 -0.928571 -0.914286 -0.9 -0.885714 -0.871429 -0.857143 -0.842857 -0.828571 -0.814286 -0.8 -0.785714 -0.771429 -0.757143 -0.742857 -0.728571 -0.714286 -0.7 -0.685714 -0.671429 -0.657143 -0.642857 -0.628571 -0.614286 -0.6 -0.585714 -0.571429 -0.557143 -0.542857 -0.528571 -0.514286 -0.5 -0.485714 -0.471429 -0.457143 -0.442857 -0.428571 -0.414286 -0.4 -0.385714 -0.371429 -0.357143 -0.342857 -0.328571 -0.314286 -0.3 -0.285714 -0.271429 -0.257143 -0.242857 -0.228571 -0.21931 -0.21931 -0.21931 -0.21931 -0.21931 -0.21931
  spline S113 degree 3 poles (44.6273, 47.2659) (44.4654, 47.1566) (44.2837, 47.08) (43.9012, 47.0007) (43.704, 46.9988) (43.3768, 47.06) (43.2458, 47.1038) (42.9992, 47.2258) (42.8849, 47.3035) (42.7828, 47.3957) knots 0 0 0 0 0.058597 0.058597 0.117193 0.117193 0.158456 0.158456 0.199718 0.199718 0.199718 0.199718
  arc A57 (42.7828, 47.3957) -> (42.664, 47.5027) centre (0, 0) ccw
  spline S114 degree 3 poles (42.664, 47.5027) (42.5187, 47.6332) (42.4003, 47.7908) (42.2305, 48.1426) (42.1808, 48.3335) (42.1607, 48.6657) (42.1714, 48.8035) (42.2299, 49.0723) (42.2776, 49.202) (42.3422, 49.3234) knots 0 0 0 0 0.058597 0.058597 0.117193 0.117193 0.158456 0.158456 0.199718 0.199718 0.199718 0.199718
  spline S115 degree 5 poles (42.3422, 49.3234) (42.3486, 49.3354) (42.3648, 49.3659) (42.3906, 49.415) (42.4259, 49.4828) (42.4704, 49.5697) (42.5176, 49.6635) (42.5642, 49.7577) (42.6103, 49.8523) (42.6559, 49.9473) (42.7009, 50.0426) (42.7454, 50.1383) (42.7893, 50.2343) (42.8327, 50.3307) (42.8756, 50.4274) (42.9181, 50.5245) (42.96, 50.6219) (43.0014, 50.7196) (43.0423, 50.8176) (43.0828, 50.9159) (43.1228, 51.0146) (43.1623, 51.1135) (43.2014, 51.2127) (43.24, 51.3122) (43.2782, 51.4119) (43.3159, 51.512) (43.3532, 51.6123) (43.3901, 51.7128) (43.4265, 51.8137) (43.4624, 51.9148) (43.498, 52.0161) (43.5331, 52.1177) (43.5678, 52.2196) (43.6021, 52.3216) (43.636, 52.424) (43.6695, 52.5265) (43.7026, 52.6293) (43.7352, 52.7324) (43.7675, 52.8356) (43.7993, 52.9391) (43.8308, 53.0428) (43.8619, 53.1467) (43.8926, 53.2509) (43.9228, 53.3552) (43.9527, 53.4598) (43.9823, 53.5646) (44.0114, 53.6696) (44.0401, 53.7748) (44.0685, 53.8801) (44.0965, 53.9857) (44.1241, 54.0915) (44.1514, 54.1975) (44.1782, 54.3037) (44.2047, 54.41) (44.2309, 54.5166) (44.2567, 54.6233) (44.277, 54.7089) (44.2921, 54.7731) (44.302, 54.8159) (44.307, 54.8374) knots 0.21931 0.21931 0.21931 0.21931 0.21931 0.21931 0.228571 0.242857 0.257143 0.271429 0.285714 0.3 0.314286 0.328571 0.342857 0.357143 0.371429 0.385714 0.4 0.414286 0.428571 0.442857 0.457143 0.471429 0.485714 0.5 0.514286 0.528571 0.542857 0.557143 0.571429 0.585714 0.6 0.614286 0.628571 0.642857 0.657143 0.671429 0.685714 0.7 0.714286 0.728571 0.742857 0.757143 0.771429 0.785714 0.8 0.814286 0.828571 0.842857 0.857143 0.871429 0.885714 0.9 0.914286 0.928571 0.942857 0.957143 0.971429 0.985714 1 1 1 1 1 1
  arc A58 (44.307, 54.8374) -> (42.4897, 56.2573) centre (0, 0) ccw
  spline S116 degree 5 poles (42.4897, 56.2573) (42.4701, 56.2473) (42.4309, 56.2272) (42.3722, 56.197) (42.2941, 56.1566) (42.1968, 56.1058) (42.0997, 56.0547) (42.0029, 56.0032) (41.9064, 55.9514) (41.8102, 55.8994) (41.7142, 55.847) (41.6185, 55.7943) (41.5231, 55.7412) (41.428, 55.6879) (41.3332, 55.6342) (41.2387, 55.5803) (41.1445, 55.5259) (41.0505, 55.4713) (40.9569, 55.4164) (40.8636, 55.3611) (40.7706, 55.3054) (40.6779, 55.2495) (40.5855, 55.1932) (40.4934, 55.1366) (40.4017, 55.0796) (40.3103, 55.0224) (40.2192, 54.9647) (40.1284, 54.9067) (40.038, 54.8484) (39.9479, 54.7898) (39.8582, 54.7307) (39.7688, 54.6714) (39.6797, 54.6117) (39.5911, 54.5516) (39.5028, 54.4911) (39.4148, 54.4303) (39.3273, 54.3692) (39.2401, 54.3076) (39.1533, 54.2457) (39.0669, 54.1834) (38.9808, 54.1207) (38.8952, 54.0577) (38.81, 53.9943) (38.7253, 53.9304) (38.6409, 53.8662) (38.557, 53.8016) (38.4735, 53.7365) (38.3905, 53.6711) (38.3079, 53.6052) (38.2258, 53.5389) (38.1442, 53.4721) (38.0631, 53.405) (37.9825, 53.3374) (37.9023, 53.2693) (37.8227, 53.2008) (37.7492, 53.1367) (37.6919, 53.086) (37.6506, 53.049) (37.6249, 53.026) (37.6148, 53.0169) knots -1 -1 -1 -1 -1 -1 -0.985714 -0.971429 -0.957143 -0.942857 -0.928571 -0.914286 -0.9 -0.885714 -0.871429 -0.857143 -0.842857 -0.828571 -0.814286 -0.8 -0.785714 -0.771429 -0.757143 -0.742857 -0.728571 -0.714286 -0.7 -0.685714 -0.671429 -0.657143 -0.642857 -0.628571 -0.614286 -0.6 -0.585714 -0.571429 -0.557143 -0.542857 -0.528571 -0.514286 -0.5 -0.485714 -0.471429 -0.457143 -0.442857 -0.428571 -0.414286 -0.4 -0.385714 -0.371429 -0.357143 -0.342857 -0.328571 -0.314286 -0.3 -0.285714 -0.271429 -0.257143 -0.242857 -0.228571 -0.21931 -0.21931 -0.21931 -0.21931 -0.21931 -0.21931
  spline S117 degree 3 poles (37.6148, 53.0169) (37.4697, 52.8861) (37.3005, 52.7849) (36.9327, 52.6532) (36.7377, 52.6238) (36.4052, 52.6389) (36.2693, 52.664) (36.0082, 52.7506) (35.8842, 52.8116) (35.7703, 52.8886) knots 0 0 0 0 0.058597 0.058597 0.117193 0.117193 0.158456 0.158456 0.199718 0.199718 0.199718 0.199718
  arc A59 (35.7703, 52.8886) -> (35.6377, 52.9781) centre (0, 0) ccw
  spline S118 degree 3 poles (35.6377, 52.9781) (35.4756, 53.0871) (35.3364, 53.2267) (35.1193, 53.5515) (35.0435, 53.7335) (34.9775, 54.0598) (34.9689, 54.1977) (34.9894, 54.472) (35.0185, 54.6071) (35.0656, 54.7363) knots 0 0 0 0 0.058597 0.058597 0.117193 0.117193 0.158456 0.158456 0.199718 0.199718 0.199718 0.199718
  spline S119 degree 5 poles (35.0656, 54.7363) (35.0703, 54.7491) (35.0821, 54.7815) (35.1008, 54.8337) (35.1264, 54.9058) (35.1583, 54.998) (35.192, 55.0975) (35.2251, 55.1973) (35.2576, 55.2973) (35.2894, 55.3977) (35.3207, 55.4984) (35.3515, 55.5993) (35.3816, 55.7006) (35.4112, 55.8021) (35.4402, 55.9038) (35.4687, 56.0059) (35.4967, 56.1081) (35.5241, 56.2106) (35.551, 56.3134) (35.5774, 56.4164) (35.6033, 56.5196) (35.6287, 56.6231) (35.6536, 56.7267) (35.678, 56.8306) (35.7019, 56.9347) (35.7253, 57.0391) (35.7483, 57.1436) (35.7708, 57.2483) (35.7928, 57.3532) (35.8143, 57.4583) (35.8354, 57.5636) (35.8561, 57.6691) (35.8763, 57.7748) (35.896, 57.8807) (35.9154, 57.9868) (35.9342, 58.093) (35.9527, 58.1994) (35.9707, 58.306) (35.9882, 58.4127) (36.0054, 58.5196) (36.0221, 58.6267) (36.0384, 58.7339) (36.0543, 58.8413) (36.0698, 58.9489) (36.0848, 59.0566) (36.0995, 59.1644) (36.1137, 59.2725) (36.1275, 59.3806) (36.141, 59.4889) (36.154, 59.5974) (36.1666, 59.706) (36.1789, 59.8147) (36.1907, 59.9236) (36.2021, 60.0326) (36.2132, 60.1418) (36.2239, 60.2511) (36.2321, 60.3386) (36.2381, 60.4043) (36.242, 60.4481) (36.2439, 60.4701) knots 0.21931 0.21931 0.21931 0.21931 0.21931 0.21931 0.228571 0.242857 0.257143 0.271429 0.285714 0.3 0.314286 0.328571 0.342857 0.357143 0.371429 0.385714 0.4 0.414286 0.428571 0.442857 0.457143 0.471429 0.485714 0.5 0.514286 0.528571 0.542857 0.557143 0.571429 0.585714 0.6 0.614286 0.628571 0.642857 0.657143 0.671429 0.685714 0.7 0.714286 0.728571 0.742857 0.757143 0.771429 0.785714 0.8 0.814286 0.828571 0.842857 0.857143 0.871429 0.885714 0.9 0.914286 0.928571 0.942857 0.957143 0.971429 0.985714 1 1 1 1 1 1
  arc A60 (36.2439, 60.4701) -> (34.2466, 61.6232) centre (0, 0) ccw
  spline S120 degree 5 poles (34.2466, 61.6232) (34.2286, 61.6105) (34.1926, 61.5852) (34.1387, 61.5472) (34.067, 61.4963) (33.9777, 61.4324) (33.8887, 61.3683) (33.8, 61.3039) (33.7117, 61.2392) (33.6236, 61.1742) (33.5359, 61.109) (33.4484, 61.0435) (33.3614, 60.9777) (33.2746, 60.9116) (33.1882, 60.8453) (33.1021, 60.7787) (33.0163, 60.7118) (32.9309, 60.6446) (32.8459, 60.5771) (32.7611, 60.5094) (32.6768, 60.4414) (32.5928, 60.3731) (32.5091, 60.3045) (32.4258, 60.2356) (32.3429, 60.1664) (32.2603, 60.097) (32.1781, 60.0272) (32.0963, 59.9572) (32.0149, 59.8869) (31.9339, 59.8162) (31.8532, 59.7453) (31.773, 59.6741) (31.6931, 59.6025) (31.6137, 59.5307) (31.5346, 59.4585) (31.456, 59.3861) (31.3778, 59.3133) (31.3, 59.2403) (31.2227, 59.1669) (31.1458, 59.0932) (31.0693, 59.0191) (30.9933, 58.9448) (30.9178, 58.8701) (30.8427, 58.7951) (30.7681, 58.7197) (30.694, 58.6441) (30.6204, 58.568) (30.5473, 58.4917) (30.4747, 58.4149) (30.4027, 58.3379) (30.3311, 58.2604) (30.2601, 58.1826) (30.1897, 58.1044) (30.1198, 58.0259) (30.0505, 57.947) (29.9867, 57.8732) (29.937, 57.8151) (29.9011, 57.7727) (29.8789, 57.7463) (29.8702, 57.7359) knots -1 -1 -1 -1 -1 -1 -0.985714 -0.971429 -0.957143 -0.942857 -0.928571 -0.914286 -0.9 -0.885714 -0.871429 -0.857143 -0.842857 -0.828571 -0.814286 -0.8 -0.785714 -0.771429 -0.757143 -0.742857 -0.728571 -0.714286 -0.7 -0.685714 -0.671429 -0.657143 -0.642857 -0.628571 -0.614286 -0.6 -0.585714 -0.571429 -0.557143 -0.542857 -0.528571 -0.514286 -0.5 -0.485714 -0.471429 -0.457143 -0.442857 -0.428571 -0.414286 -0.4 -0.385714 -0.371429 -0.357143 -0.342857 -0.328571 -0.314286 -0.3 -0.285714 -0.271429 -0.257143 -0.242857 -0.228571 -0.21931 -0.21931 -0.21931 -0.21931 -0.21931 -0.21931
  spline S121 degree 3 poles (29.8702, 57.7359) (29.7447, 57.5862) (29.5912, 57.4625) (29.2454, 57.2808) (29.0564, 57.2246) (28.725, 57.1933) (28.5869, 57.1992) (28.3163, 57.2486) (28.185, 57.2917) (28.0615, 57.3522) knots 0 0 0 0 0.058597 0.058597 0.117193 0.117193 0.158456 0.158456 0.199718 0.199718 0.199718 0.199718
  arc A61 (28.0615, 57.3522) -> (27.9178, 57.4223) centre (0, 0) ccw
  spline S122 degree 3 poles (27.9178, 57.4223) (27.7421, 57.5077) (27.5848, 57.6266) (27.3246, 57.918) (27.2242, 58.0877) (27.1134, 58.4016) (27.0857, 58.537) (27.0679, 58.8115) (27.0779, 58.9493) (27.1066, 59.0838) knots 0 0 0 0 0.058597 0.058597 0.117193 0.117193 0.158456 0.158456 0.199718 0.199718 0.199718 0.199718
  spline S123 degree 5 poles (27.1066, 59.0838) (27.1094, 59.0971) (27.1165, 59.1309) (27.1279, 59.1852) (27.1431, 59.2601) (27.1619, 59.3558) (27.1814, 59.459) (27.2003, 59.5625) (27.2185, 59.6661) (27.2361, 59.7699) (27.2531, 59.874) (27.2695, 59.9782) (27.2853, 60.0827) (27.3004, 60.1873) (27.315, 60.2921) (27.329, 60.3971) (27.3425, 60.5023) (27.3554, 60.6076) (27.3677, 60.7131) (27.3795, 60.8188) (27.3908, 60.9246) (27.4015, 61.0306) (27.4117, 61.1367) (27.4214, 61.243) (27.4306, 61.3494) (27.4393, 61.456) (27.4475, 61.5627) (27.4552, 61.6695) (27.4624, 61.7765) (27.4691, 61.8836) (27.4754, 61.9908) (27.4811, 62.0981) (27.4864, 62.2056) (27.4913, 62.3132) (27.4956, 62.4209) (27.4995, 62.5287) (27.503, 62.6366) (27.506, 62.7447) (27.5085, 62.8528) (27.5106, 62.9611) (27.5123, 63.0694) (27.5135, 63.1779) (27.5143, 63.2865) (27.5146, 63.3951) (27.5146, 63.5039) (27.5141, 63.6127) (27.5131, 63.7217) (27.5118, 63.8307) (27.51, 63.9398) (27.5078, 64.0491) (27.5052, 64.1584) (27.5022, 64.2677) (27.4987, 64.3772) (27.4949, 64.4868) (27.4906, 64.5964) (27.486, 64.7061) (27.482, 64.7939) (27.4787, 64.8598) (27.4765, 64.9038) (27.4754, 64.9257) knots 0.21931 0.21931 0.21931 0.21931 0.21931 0.21931 0.228571 0.242857 0.257143 0.271429 0.285714 0.3 0.314286 0.328571 0.342857 0.357143 0.371429 0.385714 0.4 0.414286 0.428571 0.442857 0.457143 0.471429 0.485714 0.5 0.514286 0.528571 0.542857 0.557143 0.571429 0.585714 0.6 0.614286 0.628571 0.642857 0.657143 0.671429 0.685714 0.7 0.714286 0.728571 0.742857 0.757143 0.771429 0.785714 0.8 0.814286 0.828571 0.842857 0.857143 0.871429 0.885714 0.9 0.914286 0.928571 0.942857 0.957143 0.971429 0.985714 1 1 1 1 1 1
  arc A62 (27.4754, 64.9257) -> (25.3371, 65.7897) centre (0, 0) ccw
  spline S124 degree 5 poles (25.3371, 65.7897) (25.321, 65.7747) (25.2889, 65.7446) (25.2408, 65.6994) (25.1768, 65.639) (25.0973, 65.5634) (25.0181, 65.4874) (24.9392, 65.4113) (24.8607, 65.335) (24.7826, 65.2584) (24.7048, 65.1816) (24.6273, 65.1045) (24.5502, 65.0273) (24.4735, 64.9498) (24.3972, 64.872) (24.3212, 64.7941) (24.2456, 64.7159) (24.1703, 64.6375) (24.0955, 64.5589) (24.021, 64.48) (23.947, 64.4009) (23.8733, 64.3216) (23.8, 64.242) (23.7271, 64.1622) (23.6546, 64.0822) (23.5825, 64.0019) (23.5108, 63.9214) (23.4395, 63.8406) (23.3687, 63.7597) (23.2983, 63.6784) (23.2283, 63.597) (23.1587, 63.5153) (23.0896, 63.4333) (23.0209, 63.3511) (22.9527, 63.2687) (22.8849, 63.186) (22.8176, 63.103) (22.7508, 63.0199) (22.6844, 62.9364) (22.6185, 62.8527) (22.5531, 62.7688) (22.4882, 62.6846) (22.4238, 62.6001) (22.3599, 62.5154) (22.2965, 62.4304) (22.2336, 62.3451) (22.1713, 62.2596) (22.1095, 62.1738) (22.0483, 62.0877) (21.9877, 62.0013) (21.9277, 61.9147) (21.8682, 61.8278) (21.8093, 61.7406) (21.751, 61.6531) (21.6934, 61.5653) (21.6404, 61.4833) (21.5993, 61.4188) (21.5697, 61.3719) (21.5514, 61.3426) (21.5442, 61.3311) knots -1 -1 -1 -1 -1 -1 -0.985714 -0.971429 -0.957143 -0.942857 -0.928571 -0.914286 -0.9 -0.885714 -0.871429 -0.857143 -0.842857 -0.828571 -0.814286 -0.8 -0.785714 -0.771429 -0.757143 -0.742857 -0.728571 -0.714286 -0.7 -0.685714 -0.671429 -0.657143 -0.642857 -0.628571 -0.614286 -0.6 -0.585714 -0.571429 -0.557143 -0.542857 -0.528571 -0.514286 -0.5 -0.485714 -0.471429 -0.457143 -0.442857 -0.428571 -0.414286 -0.4 -0.385714 -0.371429 -0.357143 -0.342857 -0.328571 -0.314286 -0.3 -0.285714 -0.271429 -0.257143 -0.242857 -0.228571 -0.21931 -0.21931 -0.21931 -0.21931 -0.21931 -0.21931
  spline S125 degree 3 poles (21.5442, 61.3311) (21.4408, 61.1654) (21.306, 61.0215) (20.9888, 60.7935) (20.8095, 60.7116) (20.4857, 60.6344) (20.3481, 60.6211) (20.0733, 60.6323) (19.9373, 60.6568) (19.8065, 60.6994) knots 0 0 0 0 0.058597 0.058597 0.117193 0.117193 0.158456 0.158456 0.199718 0.199718 0.199718 0.199718
  arc A63 (19.8065, 60.6994) -> (19.6544, 60.7489) centre (0, 0) ccw
  spline S126 degree 3 poles (19.6544, 60.7489) (19.4686, 60.809) (19.2963, 60.9048) (18.9981, 61.1572) (18.8751, 61.3113) (18.7216, 61.6067) (18.6753, 61.7369) (18.6195, 62.0062) (18.6102, 62.1441) (18.6199, 62.2813) knots 0 0 0 0 0.058597 0.058597 0.117193 0.117193 0.158456 0.158456 0.199718 0.199718 0.199718 0.199718
  spline S127 degree 5 poles (18.6199, 62.2813) (18.6208, 62.2949) (18.6232, 62.3293) (18.6269, 62.3847) (18.6315, 62.461) (18.6368, 62.5584) (18.6418, 62.6633) (18.6461, 62.7684) (18.6497, 62.8735) (18.6527, 62.9788) (18.655, 63.0842) (18.6568, 63.1897) (18.6578, 63.2953) (18.6583, 63.401) (18.6582, 63.5069) (18.6574, 63.6128) (18.6561, 63.7188) (18.6542, 63.8249) (18.6517, 63.9311) (18.6487, 64.0374) (18.6452, 64.1437) (18.641, 64.2502) (18.6364, 64.3567) (18.6312, 64.4633) (18.6255, 64.57) (18.6193, 64.6767) (18.6125, 64.7835) (18.6053, 64.8904) (18.5975, 64.9973) (18.5893, 65.1043) (18.5805, 65.2113) (18.5713, 65.3184) (18.5616, 65.4256) (18.5514, 65.5328) (18.5407, 65.6401) (18.5296, 65.7474) (18.518, 65.8547) (18.5059, 65.9621) (18.4934, 66.0696) (18.4804, 66.1771) (18.467, 66.2846) (18.4531, 66.3922) (18.4388, 66.4998) (18.424, 66.6075) (18.4088, 66.7152) (18.3931, 66.8229) (18.377, 66.9306) (18.3605, 67.0384) (18.3436, 67.1462) (18.3262, 67.2541) (18.3084, 67.362) (18.2902, 67.4699) (18.2715, 67.5778) (18.2525, 67.6857) (18.233, 67.7937) (18.2132, 67.9017) (18.1969, 67.9881) (18.1846, 68.0529) (18.1763, 68.0961) (18.1721, 68.1177) knots 0.21931 0.21931 0.21931 0.21931 0.21931 0.21931 0.228571 0.242857 0.257143 0.271429 0.285714 0.3 0.314286 0.328571 0.342857 0.357143 0.371429 0.385714 0.4 0.414286 0.428571 0.442857 0.457143 0.471429 0.485714 0.5 0.514286 0.528571 0.542857 0.557143 0.571429 0.585714 0.6 0.614286 0.628571 0.642857 0.657143 0.671429 0.685714 0.7 0.714286 0.728571 0.742857 0.757143 0.771429 0.785714 0.8 0.814286 0.828571 0.842857 0.857143 0.871429 0.885714 0.9 0.914286 0.928571 0.942857 0.957143 0.971429 0.985714 1 1 1 1 1 1
  arc A64 (18.1721, 68.1177) -> (15.9343, 68.6757) centre (0, 0) ccw
  spline S128 degree 5 poles (15.9343, 68.6757) (15.9205, 68.6585) (15.8929, 68.6243) (15.8515, 68.5729) (15.7966, 68.5042) (15.7284, 68.4182) (15.6605, 68.332) (15.593, 68.2456) (15.5259, 68.1591) (15.4592, 68.0723) (15.3928, 67.9855) (15.3269, 67.8984) (15.2613, 67.8111) (15.1961, 67.7237) (15.1313, 67.6361) (15.0669, 67.5484) (15.0029, 67.4604) (14.9393, 67.3723) (14.8761, 67.284) (14.8134, 67.1956) (14.751, 67.1069) (14.6891, 67.0181) (14.6276, 66.9291) (14.5665, 66.8399) (14.5059, 66.7506) (14.4456, 66.6611) (14.3859, 66.5714) (14.3265, 66.4815) (14.2676, 66.3914) (14.2092, 66.3012) (14.1512, 66.2108) (14.0937, 66.1202) (14.0367, 66.0294) (13.9801, 65.9385) (13.924, 65.8473) (13.8684, 65.756) (13.8133, 65.6645) (13.7587, 65.5728) (13.7046, 65.481) (13.651, 65.3889) (13.5979, 65.2967) (13.5453, 65.2043) (13.4933, 65.1117) (13.4418, 65.0189) (13.3909, 64.9259) (13.3405, 64.8327) (13.2907, 64.7393) (13.2415, 64.6458) (13.1928, 64.552) (13.1448, 64.4581) (13.0974, 64.3639) (13.0506, 64.2695) (13.0044, 64.175) (12.9589, 64.0802) (12.9141, 63.9852) (12.873, 63.8968) (12.8413, 63.8272) (12.8185, 63.7766) (12.8044, 63.745) (12.7989, 63.7326) knots -1 -1 -1 -1 -1 -1 -0.985714 -0.971429 -0.957143 -0.942857 -0.928571 -0.914286 -0.9 -0.885714 -0.871429 -0.857143 -0.842857 -0.828571 -0.814286 -0.8 -0.785714 -0.771429 -0.757143 -0.742857 -0.728571 -0.714286 -0.7 -0.685714 -0.671429 -0.657143 -0.642857 -0.628571 -0.614286 -0.6 -0.585714 -0.571429 -0.557143 -0.542857 -0.528571 -0.514286 -0.5 -0.485714 -0.471429 -0.457143 -0.442857 -0.428571 -0.414286 -0.4 -0.385714 -0.371429 -0.357143 -0.342857 -0.328571 -0.314286 -0.3 -0.285714 -0.271429 -0.257143 -0.242857 -0.228571 -0.21931 -0.21931 -0.21931 -0.21931 -0.21931 -0.21931
  spline S129 degree 3 poles (12.7989, 63.7326) (12.7196, 63.5542) (12.6061, 63.3929) (12.3237, 63.1229) (12.1575, 63.0168) (11.8476, 62.8954) (11.7133, 62.863) (11.4395, 62.8359) (11.3014, 62.8412) (11.166, 62.8653) knots 0 0 0 0 0.058597 0.058597 0.117193 0.117193 0.158456 0.158456 0.199718 0.199718 0.199718 0.199718
  arc A65 (11.166, 62.8653) -> (11.0086, 62.893) centre (0, 0) ccw
  spline S130 degree 3 poles (11.0086, 62.893) (10.8162, 62.9267) (10.6322, 62.9976) (10.3018, 63.206) (10.1585, 63.3415) (9.9654, 63.6127) (9.9015, 63.7352) (9.8087, 63.9941) (9.7803, 64.1294) (9.7708, 64.2666) knots 0 0 0 0 0.058597 0.058597 0.117193 0.117193 0.158456 0.158456 0.199718 0.199718 0.199718 0.199718
  spline S131 degree 5 poles (9.7708, 64.2666) (9.7698, 64.2801) (9.7674, 64.3146) (9.7633, 64.3699) (9.7573, 64.4461) (9.749, 64.5433) (9.7393, 64.6479) (9.729, 64.7525) (9.7179, 64.8572) (9.7062, 64.9618) (9.6939, 65.0665) (9.6809, 65.1713) (9.6673, 65.276) (9.653, 65.3808) (9.6381, 65.4855) (9.6227, 65.5903) (9.6066, 65.6951) (9.5899, 65.7999) (9.5727, 65.9048) (9.555, 66.0096) (9.5366, 66.1144) (9.5177, 66.2192) (9.4983, 66.3241) (9.4783, 66.4289) (9.4578, 66.5337) (9.4368, 66.6386) (9.4153, 66.7434) (9.3932, 66.8482) (9.3707, 66.953) (9.3476, 67.0578) (9.3241, 67.1626) (9.3, 67.2674) (9.2755, 67.3721) (9.2505, 67.4769) (9.225, 67.5816) (9.199, 67.6863) (9.1726, 67.791) (9.1457, 67.8957) (9.1183, 68.0004) (9.0905, 68.105) (9.0622, 68.2097) (9.0335, 68.3143) (9.0043, 68.4188) (8.9747, 68.5234) (8.9447, 68.6279) (8.9142, 68.7324) (8.8832, 68.8369) (8.8519, 68.9413) (8.8201, 69.0457) (8.7879, 69.1501) (8.7552, 69.2544) (8.7222, 69.3587) (8.6887, 69.463) (8.6548, 69.5673) (8.6205, 69.6715) (8.5858, 69.7756) (8.5577, 69.859) (8.5365, 69.9214) (8.5222, 69.9631) (8.5151, 69.9839) knots 0.21931 0.21931 0.21931 0.21931 0.21931 0.21931 0.228571 0.242857 0.257143 0.271429 0.285714 0.3 0.314286 0.328571 0.342857 0.357143 0.371429 0.385714 0.4 0.414286 0.428571 0.442857 0.457143 0.471429 0.485714 0.5 0.514286 0.528571 0.542857 0.557143 0.571429 0.585714 0.6 0.614286 0.628571 0.642857 0.657143 0.671429 0.685714 0.7 0.714286 0.728571 0.742857 0.757143 0.771429 0.785714 0.8 0.814286 0.828571 0.842857 0.857143 0.871429 0.885714 0.9 0.914286 0.928571 0.942857 0.957143 0.971429 0.985714 1 1 1 1 1 1
  arc A66 (8.5151, 69.9839) -> (6.2215, 70.2249) centre (0, 0) ccw
  spline S132 degree 5 poles (6.2215, 70.2249) (6.2101, 70.2061) (6.1875, 70.1683) (6.1538, 70.1116) (6.109, 70.036) (6.0534, 69.9413) (5.9981, 69.8465) (5.9433, 69.7516) (5.8889, 69.6565) (5.8349, 69.5614) (5.7813, 69.4661) (5.7281, 69.3707) (5.6753, 69.2752) (5.6229, 69.1795) (5.5709, 69.0838) (5.5194, 68.9879) (5.4682, 68.8919) (5.4175, 68.7958) (5.3672, 68.6996) (5.3174, 68.6032) (5.268, 68.5068) (5.219, 68.4102) (5.1705, 68.3135) (5.1224, 68.2167) (5.0748, 68.1198) (5.0276, 68.0228) (4.9809, 67.9256) (4.9347, 67.8284) (4.8889, 67.731) (4.8436, 67.6335) (4.7988, 67.5359) (4.7544, 67.4382) (4.7106, 67.3404) (4.6672, 67.2424) (4.6243, 67.1444) (4.582, 67.0462) (4.5401, 66.9479) (4.4988, 66.8495) (4.458, 66.751) (4.4177, 66.6524) (4.378, 66.5537) (4.3388, 66.4549) (4.3002, 66.3559) (4.2621, 66.2569) (4.2246, 66.1577) (4.1877, 66.0584) (4.1514, 65.959) (4.1156, 65.8595) (4.0805, 65.7599) (4.0461, 65.6602) (4.0122, 65.5603) (3.979, 65.4604) (3.9464, 65.3603) (3.9145, 65.2601) (3.8833, 65.1598) (3.855, 65.0665) (3.8333, 64.9932) (3.8178, 64.9399) (3.8082, 64.9067) (3.8045, 64.8937) knots -1 -1 -1 -1 -1 -1 -0.985714 -0.971429 -0.957143 -0.942857 -0.928571 -0.914286 -0.9 -0.885714 -0.871429 -0.857143 -0.842857 -0.828571 -0.814286 -0.8 -0.785714 -0.771429 -0.757143 -0.742857 -0.728571 -0.714286 -0.7 -0.685714 -0.671429 -0.657143 -0.642857 -0.628571 -0.614286 -0.6 -0.585714 -0.571429 -0.557143 -0.542857 -0.528571 -0.514286 -0.5 -0.485714 -0.471429 -0.457143 -0.442857 -0.428571 -0.414286 -0.4 -0.385714 -0.371429 -0.357143 -0.342857 -0.328571 -0.314286 -0.3 -0.285714 -0.271429 -0.257143 -0.242857 -0.228571 -0.21931 -0.21931 -0.21931 -0.21931 -0.21931 -0.21931
  spline S133 degree 3 poles (3.8045, 64.8937) (3.7507, 64.7059) (3.6608, 64.5304) (3.4188, 64.2238) (3.269, 64.0956) (2.979, 63.9322) (2.8504, 63.8814) (2.5831, 63.8164) (2.4457, 63.8025) (2.3082, 63.8075) knots 0 0 0 0 0.058597 0.058597 0.117193 0.117193 0.158456 0.158456 0.199718 0.199718 0.199718 0.199718
  arc A67 (2.3082, 63.8075) -> (2.1484, 63.813) centre (0, 0) ccw
  spline S134 degree 3 poles (2.1484, 63.813) (1.9532, 63.8196) (1.7611, 63.8643) (1.4049, 64.0246) (1.2442, 64.1389) (1.0153, 64.3805) (0.9349, 64.4929) (0.807, 64.7364) (0.7601, 64.8664) (0.7315, 65.001) knots 0 0 0 0 0.058597 0.058597 0.117193 0.117193 0.158456 0.158456 0.199718 0.199718 0.199718 0.199718
  spline S135 degree 5 poles (0.7315, 65.001) (0.7287, 65.0143) (0.7215, 65.048) (0.7097, 65.1022) (0.6932, 65.1769) (0.6714, 65.272) (0.6473, 65.3742) (0.6225, 65.4764) (0.597, 65.5785) (0.5708, 65.6805) (0.544, 65.7824) (0.5166, 65.8843) (0.4885, 65.9862) (0.4598, 66.0879) (0.4305, 66.1896) (0.4006, 66.2912) (0.3701, 66.3928) (0.339, 66.4942) (0.3074, 66.5956) (0.2752, 66.697) (0.2425, 66.7982) (0.2092, 66.8994) (0.1753, 67.0005) (0.141, 67.1016) (0.1061, 67.2025) (0.0707, 67.3034) (0.0348, 67.4042) (-0.0017, 67.5049) (-0.0386, 67.6056) (-0.076, 67.7061) (-0.1139, 67.8066) (-0.1523, 67.907) (-0.1912, 68.0074) (-0.2305, 68.1076) (-0.2703, 68.2078) (-0.3106, 68.3079) (-0.3514, 68.4079) (-0.3926, 68.5078) (-0.4343, 68.6076) (-0.4764, 68.7074) (-0.5189, 68.8071) (-0.5619, 68.9066) (-0.6054, 69.0061) (-0.6492, 69.1055) (-0.6936, 69.2049) (-0.7383, 69.3041) (-0.7835, 69.4032) (-0.829, 69.5023) (-0.8751, 69.6013) (-0.9215, 69.7002) (-0.9683, 69.7989) (-1.0156, 69.8976) (-1.0632, 69.9962) (-1.1113, 70.0948) (-1.1598, 70.1932) (-1.2086, 70.2915) (-1.248, 70.3701) (-1.2778, 70.429) (-1.2977, 70.4683) (-1.3077, 70.4879) knots 0.21931 0.21931 0.21931 0.21931 0.21931 0.21931 0.228571 0.242857 0.257143 0.271429 0.285714 0.3 0.314286 0.328571 0.342857 0.357143 0.371429 0.385714 0.4 0.414286 0.428571 0.442857 0.457143 0.471429 0.485714 0.5 0.514286 0.528571 0.542857 0.557143 0.571429 0.585714 0.6 0.614286 0.628571 0.642857 0.657143 0.671429 0.685714 0.7 0.714286 0.728571 0.742857 0.757143 0.771429 0.785714 0.8 0.814286 0.828571 0.842857 0.857143 0.871429 0.885714 0.9 0.914286 0.928571 0.942857 0.957143 0.971429 0.985714 1 1 1 1 1 1